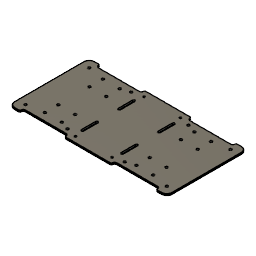
layer1_plate_v0_1 (Autodesk Fusion 360 design; units mm, degrees)
part number: 2026-05-30-11-35-53-766
Autodesk Fusion 360 part; units mm, degrees
sketch "草图1" plane through (0, 0, 0) normal (0, 1, 0) x (1, 0, 0)
  line L0 (0, 0) -> (285, 0)
  line L1 (285, 0) -> (285, -145)
  line L2 (285, -145) -> (0, -145)
  line L3 (0, -145) -> (0, 0)
  line L4 (0, -72.5) -> (285, -72.5) construction
  line L5 (142.5, 0) -> (142.5, -145) construction
  line L6 (40, -13) -> (80, -13)
  line L7 (80, -13) -> (80, -49.4)
  line L8 (77, -52.4) -> (43, -52.4)
  line L9 (40, -49.4) -> (40, -13)
  line L10 (20, 0) -> (100, 0)
  line L11 (100, 0) -> (100, -6)
  line L12 (100, -6) -> (20, -6)
  line L13 (20, -6) -> (20, 0)
  line L14 (100, -145) -> (100, -139)
  line L15 (100, -139) -> (20, -139)
  line L16 (20, -145) -> (100, -145)
  line L17 (20, -139) -> (20, -145)
  line L18 (265, -6) -> (265, 0)
  line L19 (265, 0) -> (185, 0)
  line L20 (185, -6) -> (265, -6)
  line L21 (185, 0) -> (185, -6)
  line L22 (265, -139) -> (265, -145)
  line L23 (265, -145) -> (185, -145)
  line L24 (185, -139) -> (265, -139)
  line L25 (185, -145) -> (185, -139)
  line L26 (60, -13) -> (60, 0) construction
  line L27 (183.35, -2.75) -> (101.65, -2.75)
  line L28 (101.65, -2.75) -> (101.65, -142.25)
  line L29 (101.65, -142.25) -> (183.35, -142.25)
  line L30 (183.35, -142.25) -> (183.35, -2.75)
  line L31 (183.35, -2.75) -> (101.65, -142.25) construction
  line L32 (101.65, -2.75) -> (183.35, -142.25) construction
  circle A0 centre (44.9, -20.2) radius 2.15
  circle A1 centre (44.9, -44.4) radius 2.15
  circle A2 centre (75.1, -20.2) radius 2.15
  circle A3 centre (75.1, -44.4) radius 2.15
  circle A4 centre (109.65, -134.25) radius 1.75
  circle A5 centre (175.35, -134.25) radius 1.75
  circle A6 centre (175.35, -10.75) radius 1.75
  circle A7 centre (109.65, -10.75) radius 1.75
  circle A8 centre (15, -130) radius 2.15
  circle A9 centre (270, -130) radius 2.15
  circle A10 centre (270, -15) radius 2.15
  circle A11 centre (15, -15) radius 2.15
  circle A12 centre (90.825, -15) radius 2.15
  circle A13 centre (90.825, -130) radius 2.15
  circle A14 centre (194.175, -15) radius 2.15
  circle A15 centre (194.175, -130) radius 2.15
  line L33 (108.65, -26.125) -> (108.65, -52.125)
  line L34 (104.65, -52.125) -> (104.65, -26.125)
  arc A16 (104.65, -52.125) -> (108.65, -52.125) centre (106.65, -52.125) ccw
  arc A17 (108.65, -26.125) -> (104.65, -26.125) centre (106.65, -26.125) ccw
  line L35 (104.65, -92.875) -> (104.65, -118.875)
  arc A18 (108.65, -92.875) -> (104.65, -92.875) centre (106.65, -92.875) ccw
  line L36 (108.65, -118.875) -> (108.65, -92.875)
  arc A19 (104.65, -118.875) -> (108.65, -118.875) centre (106.65, -118.875) ccw
  line L37 (180.35, -52.125) -> (180.35, -26.125)
  arc A20 (176.35, -52.125) -> (180.35, -52.125) centre (178.35, -52.125) ccw
  line L38 (176.35, -26.125) -> (176.35, -52.125)
  arc A21 (180.35, -26.125) -> (176.35, -26.125) centre (178.35, -26.125) ccw
  line L39 (176.35, -118.875) -> (176.35, -92.875)
  line L40 (180.35, -92.875) -> (180.35, -118.875)
  arc A22 (180.35, -92.875) -> (176.35, -92.875) centre (178.35, -92.875) ccw
  arc A23 (176.35, -118.875) -> (180.35, -118.875) centre (178.35, -118.875) ccw
  line L41 (60, -13) -> (60, -52.4) construction
  arc A24 (40, -49.4) -> (43, -52.4) centre (43, -49.4) ccw
  arc A25 (77, -52.4) -> (80, -49.4) centre (77, -49.4) ccw
  line L42 (245, -49.4) -> (245, -13)
  arc A26 (242, -52.4) -> (245, -49.4) centre (242, -49.4) ccw
  line L43 (208, -52.4) -> (242, -52.4)
  arc A27 (205, -49.4) -> (208, -52.4) centre (208, -49.4) ccw
  line L44 (205, -13) -> (205, -49.4)
  line L45 (245, -13) -> (205, -13)
  circle A28 centre (240.1, -20.2) radius 2.15
  circle A29 centre (209.9, -20.2) radius 2.15
  circle A30 centre (209.9, -44.4) radius 2.15
  circle A31 centre (240.1, -44.4) radius 2.15
  line L46 (40, -95.6) -> (40, -132)
  line L47 (40, -132) -> (80, -132)
  line L48 (80, -132) -> (80, -95.6)
  line L49 (77, -92.6) -> (43, -92.6)
  arc A32 (80, -95.6) -> (77, -92.6) centre (77, -95.6) ccw
  circle A33 centre (44.9, -100.6) radius 2.15
  arc A34 (43, -92.6) -> (40, -95.6) centre (43, -95.6) ccw
  circle A35 centre (75.1, -100.6) radius 2.15
  circle A36 centre (44.9, -124.8) radius 2.15
  circle A37 centre (75.1, -124.8) radius 2.15
  line L50 (205, -132) -> (205, -95.6)
  line L51 (245, -132) -> (205, -132)
  line L52 (245, -95.6) -> (245, -132)
  arc A38 (208, -92.6) -> (205, -95.6) centre (208, -95.6) ccw
  line L53 (208, -92.6) -> (242, -92.6)
  arc A39 (245, -95.6) -> (242, -92.6) centre (242, -95.6) ccw
  circle A40 centre (209.9, -100.6) radius 2.15
  circle A41 centre (240.1, -100.6) radius 2.15
  circle A42 centre (240.1, -124.8) radius 2.15
  circle A43 centre (209.9, -124.8) radius 2.15
  point P0 (40, -52.4)
  point P1 (142.5, -72.5)
  point P2 (15, -15)
  dimension "d1" = 285
  dimension "d2" = 145
  dimension "d3" = 40
  dimension "d4" = 39.4
  dimension "d5" = 80
  dimension "d6" = 6
  dimension "d7" = 7
  dimension "d8" = 60
  dimension "d11" = 81.7
  dimension "d12" = 139.5
  dimension "d31" = 4.3
  dimension "d34" = 3.5
  dimension "d35" = 8
  dimension "d36" = 8
  dimension "d41" = 4.3
  dimension "d42" = 15
  dimension "d43" = 15
  dimension "d46" = 4.3
  dimension "d47" = 10.825
  dimension "d48" = 15
  dimension "d51" = 4
  dimension "d52" = 26
  dimension "d53" = 40.75
  dimension "d54" = 3
  dimension "d57" = 8
  dimension "d58" = 30.2
  dimension "d59" = 24.2
  dimension "d60" = 3
  constraint horizontal L0
  constraint vertical L1
  constraint horizontal L2
  constraint vertical L3
  constraint coincident L0.start L3.end
  constraint midpoint L3 L4.start
  constraint midpoint L1 L4.end
  constraint midpoint L0 L5.start
  constraint midpoint L2 L5.end
  constraint horizontal L6
  constraint vertical L7
  constraint horizontal L8
  constraint vertical L9
  constraint horizontal L10
  constraint vertical L11
  constraint horizontal L12
  constraint vertical L13
  constraint symmetric L4 L10.start L16.start
  constraint symmetric L4 L10.end L14.start
  constraint symmetric L4 L11.end L14.end
  constraint symmetric L4 L12.end L15.end
  constraint symmetric L5 L10.start L18.end
  constraint symmetric L5 L10.end L19.end
  constraint symmetric L5 L11.end L20.start
  constraint symmetric L5 L12.end L18.start
  constraint symmetric L5 L14.end L24.start
  constraint symmetric L5 L14.start L23.end
  constraint symmetric L5 L15.end L22.start
  constraint symmetric L5 L16.start L22.end
  constraint midpoint L6 L26.start
  constraint coincident L0 L26.end
  constraint perpendicular L0 L26
  constraint coincident L0 L10.start
  constraint midpoint L10 L26.end
  constraint horizontal L27
  constraint perpendicular L27 L28
  constraint parallel L27 L29
  constraint parallel L28 L30
  constraint coincident L31 P1
  constraint coincident L32 P1
  constraint midpoint L4 P1
  constraint equal A0 A1
  constraint equal A0 A3
  constraint equal A0 A2
  constraint symmetric L26 A0 A2
  constraint symmetric L26 A1 A3
  constraint symmetric L5 A4 A5
  constraint symmetric L4 A5 A6
  constraint symmetric L4 A4 A7
  constraint symmetric L5 A8 A9
  constraint symmetric L4 A8.centre P2
  constraint symmetric L4 A9 A10
  constraint symmetric L4 A8 A11
  constraint symmetric L4 A12 A13
  constraint symmetric L5 A12 A14
  constraint symmetric L5 A13 A15
  constraint vertical L33
  constraint vertical L34
  constraint tangent L33 A17
  constraint tangent L33 A16
  constraint symmetric L4 L34.end L35.end
  constraint symmetric L4 L33.start L36.start
  constraint symmetric L4 L33.end A18.start
  constraint symmetric L4 L34.start L35.start
  constraint symmetric L4 A16 A18
  constraint symmetric L4 A17 A19
  constraint symmetric L5 L34.end L37.end
  constraint symmetric L5 L33.start L38.start
  constraint symmetric L5 L33.end A20.start
  constraint symmetric L5 L34.start L37.start
  constraint symmetric L5 A16 A20
  constraint symmetric L5 A17 A21
  constraint symmetric L5 L35.start L40.start
  constraint symmetric L5 L35.end L40.end
  constraint symmetric L5 A18.start L39.end
  constraint symmetric L5 A18 A22
  constraint symmetric L5 L36.start L39.start
  constraint symmetric L5 A19 A23
  constraint tangent L34 A16
  constraint tangent L34 A17
  constraint symmetric A1 A3 L41
  constraint symmetric A0 A2 L41
  constraint coincident L8 L41.end
  constraint coincident P0 L9
  constraint coincident P0 L8
  constraint tangent L9 A24
  constraint tangent L8 A24
  constraint tangent L8 A25
  constraint tangent L7 A25
  constraint equal A24 A25
  constraint symmetric L5 L6.start L42.end
  constraint symmetric L5 L6.end L44.start
  constraint symmetric L5 A0 A28
  constraint symmetric L5 A1 A31
  constraint symmetric L5 A2 A29
  constraint symmetric L5 A3 A30
  constraint symmetric L5 L9.start L42.start
  constraint symmetric L5 L8.end A26.start
  constraint symmetric L5 A24 A26
  constraint symmetric L5 L8.start L43.start
  constraint symmetric L5 L7.end A27.start
  constraint symmetric L5 A25 A27
  constraint symmetric L4 L6.start L46.end
  constraint symmetric L4 L6.end L47.end
  constraint symmetric L4 A0 A36
  constraint symmetric L4 A1 A33
  constraint symmetric L4 A2 A37
  constraint symmetric L4 A3 A35
  constraint symmetric L4 L9.start L46.start
  constraint symmetric L4 L8.end L49.end
  constraint symmetric L4 A24 A34
  constraint symmetric L4 L8.start L49.start
  constraint symmetric L4 L7.end L48.end
  constraint symmetric L4 A25 A32
  constraint symmetric L4 L42.start L52.start
  constraint symmetric L4 L42.end L51.start
  constraint symmetric L4 A26.start L53.end
  constraint symmetric L4 A26 A39
  constraint symmetric L4 L43.start A38.start
  constraint symmetric L4 A27.start L50.end
  constraint symmetric L4 A27 A38
  constraint symmetric L4 L44.start L50.start
  constraint symmetric L4 A28 A42
  constraint symmetric L4 A29 A43
  constraint symmetric L4 A30 A40
  constraint symmetric L4 A31 A41
  measures "d1" distance of L0.start L0.end
  measures "d2" distance of L0.start L2.end
  measures "d3" distance of L6.start L6.end
  measures "d4" distance of L6.start P0
  measures "d5" distance of L10.start L10.end
  measures "d6" distance of L10.start L12.end
  measures "d7" distance of L6 L12
  measures "d8" distance of L0.start L26.end
  measures "d11" distance of L28.end L29.end
  measures "d12" distance of L27.end L28.end
  measures "d31" diameter of A0
  measures "d34" diameter of A4
  measures "d35" distance of L29 A4.centre
  measures "d36" distance of L28 A4.centre
  measures "d41" diameter of A8
  measures "d42" distance of L2 A8.centre
  measures "d43" distance of L3 A8.centre
  measures "d46" diameter of A12
  measures "d47" distance of L28 A12.centre
  measures "d48" distance of L0 A12.centre
  measures "d51" distance of L34.end L33.start
  measures "d52" distance of L34.end L34.start
  measures "d53" distance of A16.centre A18.centre
  measures "d54" distance of L28 L34
  measures "d57" distance of L8 A1.centre
  measures "d58" distance of A1.centre A3.centre
  measures "d59" distance of A0.centre A1.centre
  measures "d60" radius of A24
extrude "拉伸1" add sketch "草图1" along normal blind 3 contours L0 L1 L2 L3 L11 L12 L13 L14 L15 L17 L18 L20 L21 L22 L24 L25 | L6 L7 L8 L9 A24 A25 | L27 L28 L29 L30 | A0 | A1 | A2 | A3 | A4 | A5 | A6 | A7 | A8 | A9 | A10 | A11 | A12 | A13 | A14 | A15 | L33 L34 A16 A17 | L35 A18 L36 A19 | L37 A20 L38 A21 | L39 L40 A22 A23 | L42 A26 L43 A27 L44 L45 | A28 | A29 | A30 | A31 | L46 L47 L48 L49 A32 A34 | A33 | A35 | A36 | A37 | L50 L51 L52 A38 L53 A39 | A40 | A41 | A42 | A43
fillet "圆角1" radius 10 1 edges at (0, 1.5, 145)
fillet "圆角2" radius 10 1 edges at (0, 1.5, 0)
fillet "圆角3" radius 10 1 edges at (285, 1.5, 145)
fillet "圆角4" radius 10 1 edges at (285, 1.5, 0)
fillet "圆角5" radius 3 1 edges at (265, 1.5, 0)
fillet "圆角6" radius 3 1 edges at (265, 1.5, 6)
fillet "圆角7" radius 3 6 edges at (185, 1.5, 6) (185, 1.5, 0) (100, 1.5, 0) (100, 1.5, 6) (20, 1.5, 0) (20, 1.5, 6)
fillet "圆角8" radius 3 4 edges at (185, 1.5, 145) (185, 1.5, 139) (265, 1.5, 145) (265, 1.5, 139)
fillet "圆角9" radius 3 4 edges at (20, 1.5, 145) (20, 1.5, 139) (100, 1.5, 139) (100, 1.5, 145)
extrude "拉伸2" cut sketch "草图1" along normal blind 4 contours A0 | A1 | A2 | A3 | A4 | A5 | A6 | A7
fillet "圆角10" radius 0.5 64 edges at (184.1213, 0, 0.8787) (185.8787, 0, 5.1213) (225, 0, 6) (264.1213, 0, 5.1213) (265.8787, 0, 0.8787) (271.5, 0, 0) (282.0711, 0, 2.9289) (285, 0, 72.5) (282.0711, 0, 142.0711) (271.5, 0, 145) (265.8787, 0, 144.1213) (264.1213, 0, 139.8787) (225, 0, 139) (185.8787, 0, 139.8787) (184.1213, 0, 144.1213) (142.5, 0, 145) (100.8787, 0, 144.1213) (99.1213, 0, 139.8787) (60, 0, 139) (20.8787, 0, 139.8787) (19.1213, 0, 144.1213) (13.5, 0, 145) (2.9289, 0, 142.0711) (0, 0, 72.5) (2.9289, 0, 2.9289) (13.5, 0, 0) (19.1213, 0, 0.8787) (20.8787, 0, 5.1213) (60, 0, 6) (99.1213, 0, 5.1213) (100.8787, 0, 0.8787) (142.5, 0, 0) (185.8787, 3, 5.1213) (184.1213, 3, 0.8787) (142.5, 3, 0) (100.8787, 3, 0.8787) (99.1213, 3, 5.1213) (60, 3, 6) (20.8787, 3, 5.1213) (19.1213, 3, 0.8787) (13.5, 3, 0) (2.9289, 3, 2.9289) (0, 3, 72.5) (2.9289, 3, 142.0711) (13.5, 3, 145) (19.1213, 3, 144.1213) (20.8787, 3, 139.8787) (60, 3, 139) (99.1213, 3, 139.8787) (100.8787, 3, 144.1213) (142.5, 3, 145) (184.1213, 3, 144.1213) (185.8787, 3, 139.8787) (225, 3, 139) (264.1213, 3, 139.8787) (265.8787, 3, 144.1213) (271.5, 3, 145) (282.0711, 3, 142.0711) (285, 3, 72.5) (282.0711, 3, 2.9289) (271.5, 3, 0) (265.8787, 3, 0.8787) (264.1213, 3, 5.1213) (225, 3, 6)
extrude "拉伸3" cut sketch "草图1" along normal blind 4 contours A8 | A9 | A10 | A11
extrude "拉伸4" cut sketch "草图1" along normal blind 4 contours A12 | A13 | A14 | A15
extrude "拉伸5" cut sketch "草图1" along normal blind 4 contours L33 L34 A16 A17 | L35 A18 L36 A19 | L37 A20 L38 A21 | L39 L40 A22 A23
extrude "拉伸6" cut sketch "草图1" along normal blind 3 contours A28 | A29 | A30 | A31 | A33 | A35 | A36 | A37 | A40 | A41 | A42 | A43
